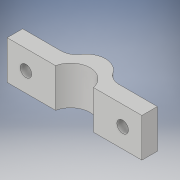
# Autodesk Inventor part: Klemme
Saved by Autodesk Inventor 2017 (Build 210142000, 142)
## iProperties
Part Number: Klemme
Material: Generisch
Document SubType Name: Modeling
Designer: pgmadmin
Density: 1 g/cm^3
Appearance: Vorgabe
Author: pgmadmin
Autodesk Inventor part; units mm, degrees
ref_plane "YZ Plane" through (0, 0, 0) normal (1, 0, 0) x (0, 1, 0)
ref_plane "XZ Plane" through (0, 0, 0) normal (0, 1, 0) x (-1, 0, 0)
ref_plane "XY Plane" through (0, 0, 0) normal (0, 0, 1) x (1, 0, 0)
sketch "Skizze1" plane through (0, 0, 0) normal (0, 0, 1) x (1, 0, 0)
  arc A0 (4.899, 1) -> (-4.899, 1) centre (0, 0) ccw
  line L0 (-17.399, 1) -> (-7.218, 1)
  line L1 (-7.218, 1) -> (-4.899, 1)
  line L2 (4.899, 1) -> (17.399, 1)
  line L3 (17.399, 1) -> (17.399, -3)
  line L4 (-17.399, -3) -> (-17.399, 1)
  arc A1 (4.899, -3) -> (-4.899, -3) centre (0, -4) ccw
  line L5 (17.399, -3) -> (4.899, -3)
  line L6 (-4.899, -3) -> (-17.399, -3)
  dimension "d0" = 10
  dimension "d1" = 1
  dimension "d3" = 10
  dimension "d16" = 4
  dimension "d17" = 12.5
  dimension "d18" = 12.5
  constraints: 14 end point, 5 perpendicular, 4 point on circle, 2 centre point, 2 horizontal, 2 point on line, 1 coincident
  measures "d0" diameter of A0
  measures "d1" distance from line of point (0, 0) L0
  measures "d3" diameter of A1
  measures "d16" distance between parallel lines of L0 L6
  measures "d17" distance from line of L4 L1.end
  measures "d18" distance of L2.end L2.start
extrude "Extrusion1" add sketch "Skizze1" along normal blind 10
fillet "Rundung1" radius 4 2 edges at (-4.899, 1, 5) (4.899, 1, 5)
sketch "Skizze4" plane through (-17.399, 1, 10) normal (0, 1, 0) x (1, 0, 0)
  line L0 (0, 10) -> (9.9157, 10) projected
  line L1 (0, 10) -> (0, 0) projected
  line L2 (9.9157, 0) -> (0, 0) projected
  line L3 (9.9157, 10) -> (9.9157, 0) projected
  line L4 (34.798, 10) -> (34.798, 0) projected
  line L5 (24.8823, 10) -> (34.798, 10) projected
  line L6 (24.8823, 0) -> (24.8823, 10) projected
  line L7 (34.798, 0) -> (24.8823, 0) projected
  point P0 (17.399, 10)
  point P1 (4.8401, 5)
  point P2 (29.8401, 5)
  dimension "d19" = 25
  measures "d19" distance of point (29.84, 5) point (4.84, 5)
hole "Bohrung2" at (-12.5589, 1, 5) at (12.4411, 1, 5) direction (0, -1, 0) diameter 3 end through all
